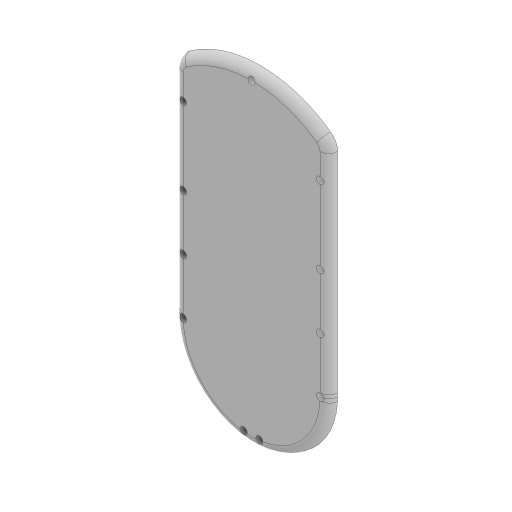
# Autodesk Inventor part: top plate
Saved by Autodesk Inventor 2024 (Build 280153000, 153)
## iProperties
Created: 2024-08-03
Part Number: top plate
Material: Generic
Document SubType Name: Modeling
Designer: chris
Density: 1 g/cm^3
Appearance: Default
Author: chris
Autodesk Inventor part; units mm, degrees
ref_plane "YZ Plane" through (0, 0, 0) normal (1, 0, 0) x (0, 1, 0)
ref_plane "XZ Plane" through (0, 0, 0) normal (0, 1, 0) x (-1, 0, 0)
ref_plane "XY Plane" through (0, 0, 0) normal (0, 0, 1) x (1, 0, 0)
sketch "Sketch1" plane through (0, 0, 0) normal (0, 0, 1) x (1, 0, 0)
  arc A0 (44.4535, 146.578395) -> (40.442974, 154.344746) centre (34.9285, 146.578395) ccw
  arc A1 (40.442974, 154.344746) -> (-40.435974, 154.344746) centre (0.0035, 97.391506) ccw
  arc A2 (-40.435974, 154.344746) -> (-44.4465, 146.578395) centre (-34.9215, 146.578395) ccw
  line L0 (-44.4465, 146.578395) -> (-44.4465, 24.273043)
  arc A3 (-44.4465, 24.273043) -> (44.4535, 24.273043) centre (0.0035, 24.273043) ccw
  line L1 (44.4535, 24.273043) -> (44.4535, 146.578395)
  circle A4 centre (-4.5, -14.5) radius 2
  circle A5 centre (-39.3665, 24.273043) radius 2
  circle A6 centre (39.3735, 24.273043) radius 2
  circle A7 centre (4.5, -14.5) radius 2
  circle A8 centre (-39.3665, 56.023043) radius 2
  circle A9 centre (-39.3665, 87.773043) radius 2
  circle A10 centre (-39.3665, 132.223043) radius 2
  circle A11 centre (0.0035, 162.161506) radius 2
  circle A12 centre (39.3735, 56.023043) radius 2
  circle A13 centre (39.3735, 87.773043) radius 2
  circle A14 centre (39.3735, 132.223043) radius 2
  point P0 (0, 0)
  point P1 (0, 0)
  constraints: 15 centre point, 8 point on circle, 4 end point
extrude "Extrusion1" add sketch "Sketch1" along normal blind 5.08
fillet "Fillet1" radius 5.08 6 edges at (-43.3847, 150.9488, 5.08) (-44.4465, 85.4257, 5.08) (0.0035, -20.177, 5.08) (44.4535, 85.4257, 5.08) (43.3917, 150.9488, 5.08) (0.0035, 167.2415, 5.08)
body "Solid1"
